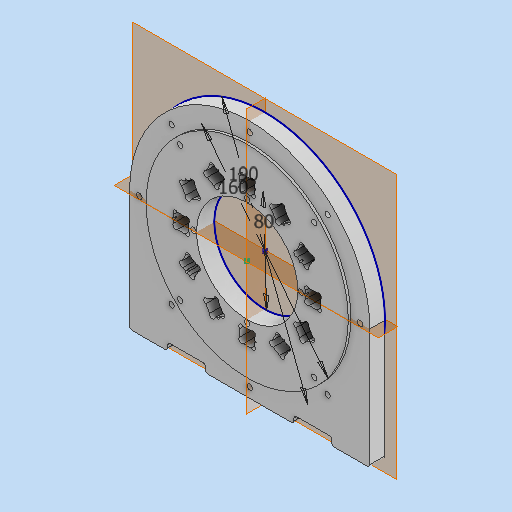
# Autodesk Inventor part: Ring 42 final
Saved by Autodesk Inventor 2026 (Build 300175050, 175E)
## iProperties
Created: 2025-09-01
Part Number: Ring 42 final
Material: Generic
Document SubType Name: Modeling
Designer: user
Density: 1 g/cm^3
Appearance: Default
Author: user
Autodesk Inventor part; units mm, degrees
sketch "Block1" plane through (0, 0, 0) normal (0, 0, 1) x (1, 0, 0)
  line L0 (58.086, -5.94) -> (46.206, -5.94)
  line L1 (46.206, -5.94) -> (46.206, 5.94)
  line L2 (46.206, 5.94) -> (58.086, 5.94)
  line L3 (58.086, 5.94) -> (58.086, -5.94)
  circle A0 centre (47.619, -4.527) radius 2.1
  circle A1 centre (47.619, 4.527) radius 2.1
  circle A2 centre (56.673, 4.527) radius 2.1
  circle A3 centre (56.673, -4.527) radius 2.1
  circle A4 centre (52.146, 0) radius 2
  circle A5 centre (45.846, 0) radius 0.75
  line L4 (45.846, 0) -> (52.146, 0)
  point P0 (52.146, 0)
  dimension "d10" = 4.2
  dimension "d11" = 4.2
  dimension "d12" = 4.2
  dimension "d13" = 4.2
  dimension "d8" = 11.88
  dimension "d9" = 11.88
  dimension "d15" = 1.413
  dimension "d16" = 1.413
  dimension "d17" = 1.413
  dimension "d18" = 1.413
  dimension "d19" = 4
  dimension "d24" = 4.527
  dimension "d25" = 4.527
  dimension "d26" = 1.5
  dimension "d27" = 6.3
  measures "d8" distance of point (46.206, 5.94) point (58.086, 5.94)
  measures "d9" distance of point (58.086, 5.94) point (58.086, -5.94)
  measures "d19" diameter of A4
  measures "d24" horizontal distance of point (56.673, 4.527) L4.end
  measures "d25" horizontal distance of point (47.619, 4.527) L4.end
  measures "d26" diameter of A5
  measures "d27" distance of L4.end L4.start
sketch "Sketch1" plane through (0, 0, 0) normal (0, 0, 1) x (1, 0, 0)
  circle A0 centre (0, 0) radius 40
  circle A1 centre (0, 0) radius 80
  circle A2 centre (0, 0) radius 95
  dimension "d0" = 80
  dimension "d1" = 160
  dimension "d2" = 190
  constraints: 3 centre point, 3 coincident
  measures "d0" diameter of A0
  measures "d1" diameter of A1
  measures "d2" diameter of A2
extrude "Extrusion1" add sketch "Sketch1" along normal blind 14 contours A1
extrude "Extrusion2" add sketch "Sketch1" along normal blind 12 contours A2
sketch "Sketch2" plane through (0, 0, 0) normal (0, 1, 0) x (-1, 0, 0)
  point P0 (0, 0)
sketch "Sketch3" plane through (0, 0, 14) normal (0, 0, 1) x (1, 0, 0)
  point P0 (0, 0)
sketch "Sketch4" plane through (0, 0, 14) normal (0, 0, 1) x (1, 0, 0)
  circle A0 centre (0, 0) radius 52.146
  line L0 (58.086, -5.94) -> (46.206, 5.94) construction
  line L1 (46.206, -5.94) -> (58.086, 5.94) construction
  line L2 (0, 0) -> (52.146, 0)
  line L3 (0, 0) -> (45.1598, 26.073)
  line L4 (0, 0) -> (26.073, 45.1598)
  line L5 (0, 0) -> (0, 52.146)
  line L6 (0, 0) -> (-26.073, 45.1598)
  line L7 (0, 0) -> (-45.1598, 26.073)
  line L8 (0, 0) -> (-52.146, 0)
  line L9 (0, 0) -> (-45.1598, -26.073)
  line L10 (0, 0) -> (-26.073, -45.1598)
  line L11 (0, 0) -> (0, -52.146)
  line L12 (0, 0) -> (26.073, -45.1598)
  line L13 (0, 0) -> (45.1598, -26.073)
  line L14 (58.086, -5.94) -> (46.206, -5.94)
  line L15 (46.206, -5.94) -> (46.206, 5.94)
  line L16 (46.206, 5.94) -> (58.086, 5.94)
  line L17 (58.086, 5.94) -> (58.086, -5.94)
  circle A1 centre (47.619, -4.527) radius 2.1
  circle A2 centre (47.619, 4.527) radius 2.1
  circle A3 centre (56.673, 4.527) radius 2.1
  circle A4 centre (56.673, -4.527) radius 2.1
  circle A5 centre (52.146, 0) radius 2
  circle A6 centre (45.846, 0) radius 0.75
  line L18 (45.846, 0) -> (52.146, 0)
  line L19 (58.086, -5.94) -> (46.206, -5.94)
  line L20 (46.206, -5.94) -> (46.206, 5.94)
  line L21 (46.206, 5.94) -> (58.086, 5.94)
  line L22 (58.086, 5.94) -> (58.086, -5.94)
  circle A7 centre (47.619, -4.527) radius 2.1
  circle A8 centre (47.619, 4.527) radius 2.1
  circle A9 centre (56.673, 4.527) radius 2.1
  circle A10 centre (56.673, -4.527) radius 2.1
  circle A11 centre (52.146, 0) radius 2
  circle A12 centre (45.846, 0) radius 0.75
  line L23 (45.846, 0) -> (52.146, 0)
  line L24 (53.274, 28.2472) -> (47.334, 17.9588)
  line L25 (47.334, 17.9588) -> (37.0456, 23.8988)
  line L26 (37.0456, 23.8988) -> (42.9856, 34.1872)
  line L27 (42.9856, 34.1872) -> (53.274, 28.2472)
  circle A13 centre (46.8168, 19.889) radius 2.1
  circle A14 centre (38.9758, 24.416) radius 2.1
  circle A15 centre (43.5028, 32.257) radius 2.1
  circle A16 centre (51.3438, 27.73) radius 2.1
  circle A17 centre (45.1598, 26.073) radius 2
  circle A18 centre (42.0098, 20.617) radius 0.75
  line L28 (42.0098, 20.617) -> (45.1598, 26.073)
  line L29 (28.2472, 53.274) -> (34.1872, 42.9856)
  line L30 (34.1872, 42.9856) -> (23.8988, 37.0456)
  line L31 (23.8988, 37.0456) -> (17.9588, 47.334)
  line L32 (17.9588, 47.334) -> (28.2472, 53.274)
  circle A19 centre (32.257, 43.5028) radius 2.1
  circle A20 centre (24.416, 38.9758) radius 2.1
  circle A21 centre (19.889, 46.8168) radius 2.1
  circle A22 centre (27.73, 51.3438) radius 2.1
  circle A23 centre (26.073, 45.1598) radius 2
  circle A24 centre (29.223, 39.7038) radius 0.75
  line L33 (29.223, 39.7038) -> (26.073, 45.1598)
  line L34 (-5.94, 58.086) -> (5.94, 58.086)
  line L35 (5.94, 58.086) -> (5.94, 46.206)
  line L36 (5.94, 46.206) -> (-5.94, 46.206)
  line L37 (-5.94, 46.206) -> (-5.94, 58.086)
  circle A25 centre (4.527, 56.673) radius 2.1
  circle A26 centre (4.527, 47.619) radius 2.1
  circle A27 centre (-4.527, 47.619) radius 2.1
  circle A28 centre (-4.527, 56.673) radius 2.1
  circle A29 centre (0, 52.146) radius 2
  circle A30 centre (6.3, 52.146) radius 0.75
  line L38 (6.3, 52.146) -> (0, 52.146)
  line L39 (-34.1872, 42.9856) -> (-28.2472, 53.274)
  line L40 (-28.2472, 53.274) -> (-17.9588, 47.334)
  line L41 (-17.9588, 47.334) -> (-23.8988, 37.0456)
  line L42 (-23.8988, 37.0456) -> (-34.1872, 42.9856)
  circle A31 centre (-27.73, 51.3438) radius 2.1
  circle A32 centre (-19.889, 46.8168) radius 2.1
  circle A33 centre (-24.416, 38.9758) radius 2.1
  circle A34 centre (-32.257, 43.5028) radius 2.1
  circle A35 centre (-26.073, 45.1598) radius 2
  circle A36 centre (-22.923, 50.6157) radius 0.75
  line L43 (-22.923, 50.6157) -> (-26.073, 45.1598)
  line L44 (-47.334, 17.9588) -> (-53.274, 28.2472)
  line L45 (-53.274, 28.2472) -> (-42.9856, 34.1872)
  line L46 (-42.9856, 34.1872) -> (-37.0456, 23.8988)
  line L47 (-37.0456, 23.8988) -> (-47.334, 17.9588)
  circle A37 centre (-51.3438, 27.73) radius 2.1
  circle A38 centre (-43.5028, 32.257) radius 2.1
  circle A39 centre (-38.9758, 24.416) radius 2.1
  circle A40 centre (-46.8168, 19.889) radius 2.1
  circle A41 centre (-45.1598, 26.073) radius 2
  circle A42 centre (-48.3098, 31.529) radius 0.75
  line L48 (-48.3098, 31.529) -> (-45.1598, 26.073)
  line L49 (-37.0456, -23.8988) -> (-42.9856, -34.1872)
  line L50 (-42.9856, -34.1872) -> (-53.274, -28.2472)
  line L51 (-53.274, -28.2472) -> (-47.334, -17.9588)
  line L52 (-47.334, -17.9588) -> (-37.0456, -23.8988)
  circle A43 centre (-43.5028, -32.257) radius 2.1
  circle A44 centre (-51.3438, -27.73) radius 2.1
  circle A45 centre (-46.8168, -19.889) radius 2.1
  circle A46 centre (-38.9758, -24.416) radius 2.1
  circle A47 centre (-45.1598, -26.073) radius 2
  circle A48 centre (-48.3098, -31.529) radius 0.75
  line L53 (-48.3098, -31.529) -> (-45.1598, -26.073)
  line L54 (-23.8988, -37.0456) -> (-17.9588, -47.334)
  line L55 (-17.9588, -47.334) -> (-28.2472, -53.274)
  line L56 (-28.2472, -53.274) -> (-34.1872, -42.9856)
  line L57 (-34.1872, -42.9856) -> (-23.8988, -37.0456)
  circle A49 centre (-19.889, -46.8168) radius 2.1
  circle A50 centre (-27.73, -51.3438) radius 2.1
  circle A51 centre (-32.257, -43.5028) radius 2.1
  circle A52 centre (-24.416, -38.9758) radius 2.1
  circle A53 centre (-26.073, -45.1598) radius 2
  circle A54 centre (-22.923, -50.6157) radius 0.75
  line L58 (-22.923, -50.6157) -> (-26.073, -45.1598)
  line L59 (17.9588, -47.334) -> (23.8988, -37.0456)
  line L60 (23.8988, -37.0456) -> (34.1872, -42.9856)
  line L61 (34.1872, -42.9856) -> (28.2472, -53.274)
  line L62 (28.2472, -53.274) -> (17.9588, -47.334)
  circle A55 centre (24.416, -38.9758) radius 2.1
  circle A56 centre (32.257, -43.5028) radius 2.1
  circle A57 centre (27.73, -51.3438) radius 2.1
  circle A58 centre (19.889, -46.8168) radius 2.1
  circle A59 centre (26.073, -45.1598) radius 2
  circle A60 centre (29.223, -39.7038) radius 0.75
  line L63 (29.223, -39.7038) -> (26.073, -45.1598)
  line L64 (42.9856, -34.1872) -> (37.0456, -23.8988)
  line L65 (37.0456, -23.8988) -> (47.334, -17.9588)
  line L66 (47.334, -17.9588) -> (53.274, -28.2472)
  line L67 (53.274, -28.2472) -> (42.9856, -34.1872)
  circle A61 centre (38.9758, -24.416) radius 2.1
  circle A62 centre (46.8168, -19.889) radius 2.1
  circle A63 centre (51.3438, -27.73) radius 2.1
  circle A64 centre (43.5028, -32.257) radius 2.1
  circle A65 centre (45.1598, -26.073) radius 2
  circle A66 centre (42.0098, -20.617) radius 0.75
  line L68 (42.0098, -20.617) -> (45.1598, -26.073)
  line L69 (-5.94, -46.206) -> (5.94, -46.206)
  line L70 (5.94, -46.206) -> (5.94, -58.086)
  line L71 (5.94, -58.086) -> (-5.94, -58.086)
  line L72 (-5.94, -58.086) -> (-5.94, -46.206)
  circle A67 centre (4.527, -47.619) radius 2.1
  circle A68 centre (4.527, -56.673) radius 2.1
  circle A69 centre (-4.527, -56.673) radius 2.1
  circle A70 centre (-4.527, -47.619) radius 2.1
  circle A71 centre (0, -52.146) radius 2
  circle A72 centre (6.3, -52.146) radius 0.75
  line L73 (6.3, -52.146) -> (0, -52.146)
  line L74 (-46.206, -5.94) -> (-58.086, -5.94)
  line L75 (-58.086, -5.94) -> (-58.086, 5.94)
  line L76 (-58.086, 5.94) -> (-46.206, 5.94)
  line L77 (-46.206, 5.94) -> (-46.206, -5.94)
  circle A73 centre (-56.673, -4.527) radius 2.1
  circle A74 centre (-56.673, 4.527) radius 2.1
  circle A75 centre (-47.619, 4.527) radius 2.1
  circle A76 centre (-47.619, -4.527) radius 2.1
  circle A77 centre (-52.146, 0) radius 2
  circle A78 centre (-58.446, 0) radius 0.75
  line L78 (-58.446, 0) -> (-52.146, 0)
  point P0 (52.146, 0)
  point P1 (-22.4156, -39.6147)
  point P2 (-26.4679, -38.5288)
  point P3 (-31.6181, -41.5023)
  point P4 (-32.7039, -45.5547)
  point P5 (-29.7305, -50.7049)
  point P6 (-25.6781, -51.7907)
  point P7 (-20.5279, -48.8172)
  point P8 (-19.4421, -44.7649)
  point P9 (-2.9735, -46.206)
  point P10 (-5.94, -49.1725)
  point P11 (-5.94, -55.1195)
  point P12 (-2.9735, -58.086)
  point P13 (2.9735, -58.086)
  point P14 (5.94, -55.1195)
  point P15 (5.94, -49.1725)
  point P16 (2.9735, -46.206)
  point P17 (31.6181, -41.5023)
  point P18 (26.4679, -38.5288)
  point P19 (22.4156, -39.6147)
  point P20 (19.4421, -44.7649)
  point P21 (20.5279, -48.8172)
  point P22 (25.6781, -51.7907)
  point P23 (29.7305, -50.7049)
  point P24 (32.7039, -45.5547)
  point P25 (39.6147, -22.4156)
  point P26 (38.5288, -26.4679)
  point P27 (41.5023, -31.6181)
  point P28 (45.5547, -32.7039)
  point P29 (50.7049, -29.7305)
  point P30 (51.7907, -25.6781)
  point P31 (48.8172, -20.5279)
  point P32 (44.7649, -19.4421)
  point P33 (49.1725, 5.94)
  point P34 (46.206, 2.9735)
  point P35 (46.206, -2.9735)
  point P36 (49.1725, -5.94)
  point P37 (55.1195, -5.94)
  point P38 (58.086, -2.9735)
  point P39 (58.086, 2.9735)
  point P40 (55.1195, 5.94)
  point P41 (39.6147, 22.4156)
  point P42 (44.7649, 19.4421)
  point P43 (48.8172, 20.5279)
  point P44 (51.7907, 25.6781)
  point P45 (50.7049, 29.7305)
  point P46 (45.5547, 32.7039)
  point P47 (41.5023, 31.6181)
  point P48 (38.5288, 26.4679)
  point P49 (20.5279, 48.8172)
  point P50 (19.4421, 44.7649)
  point P51 (22.4156, 39.6147)
  point P52 (26.4679, 38.5288)
  point P53 (31.6181, 41.5023)
  point P54 (32.7039, 45.5547)
  point P55 (29.7305, 50.7049)
  point P56 (25.6781, 51.7907)
  point P57 (-5.94, 49.1725)
  point P58 (-2.9735, 46.206)
  point P59 (2.9735, 46.206)
  point P60 (5.94, 49.1725)
  point P61 (5.94, 55.1195)
  point P62 (2.9735, 58.086)
  point P63 (-2.9735, 58.086)
  point P64 (-5.94, 55.1195)
  point P65 (-20.5279, 48.8172)
  point P66 (-25.6781, 51.7907)
  point P67 (-29.7305, 50.7049)
  point P68 (-32.7039, 45.5547)
  point P69 (-31.6181, 41.5023)
  point P70 (-26.4679, 38.5288)
  point P71 (-22.336, 38.687)
  point P72 (-22.6435, 39.2198)
  point P73 (-19.4421, 44.7649)
  point P74 (-44.7649, 19.4421)
  point P75 (-39.6147, 22.4156)
  point P76 (-38.5288, 26.4679)
  point P77 (-41.5023, 31.6181)
  point P78 (-45.5547, 32.7039)
  point P79 (-50.7049, 29.7305)
  point P80 (-51.7907, 25.6781)
  point P81 (-48.8172, 20.5279)
  point P82 (-49.1725, -5.94)
  point P83 (-46.206, -2.9735)
  point P84 (-46.206, 2.9735)
  point P85 (-49.1725, 5.94)
  point P86 (-55.1195, 5.94)
  point P87 (-58.086, 2.9735)
  point P88 (-58.086, -2.9735)
  point P89 (-55.1195, -5.94)
  point P90 (-48.8172, -20.5279)
  point P91 (-51.7907, -25.6781)
  point P92 (-50.7049, -29.7305)
  point P93 (-48.6996, -30.8882)
  point P94 (-47.56, -31.5462)
  point P95 (-45.5547, -32.7039)
  point P96 (-41.5314, -31.5333)
  point P97 (-41.487, -31.5917)
  point P98 (-38.5288, -26.4679)
  point P99 (-39.6147, -22.4156)
  point P100 (-44.7649, -19.4421)
  dimension "d7" = 104.292
  dimension "d28" = 52.146
  dimension "d31" = 360
  dimension "d33" = 0
  dimension "d34" = -60
  dimension "d35" = -120
  dimension "d36" = -180
  dimension "d37" = -180
  dimension "d38" = -240
  dimension "d39" = -300
  dimension "d40" = -60
  dimension "d41" = -120
  dimension "d42" = -180
  dimension "d43" = -240
  dimension "d44" = -240
  constraints: 28 end point, 2 midpoint, 1 centre point, 1 coincident, 1 horizontal, 57 other
  measures "d7" diameter of A0
  measures "d28" distance of point (52.146, 0) point (0, 0)
  measures "d33" vertical extent of L2
  measures "d36" angle to the sketch x axis of L2
  measures "d37" angle to the sketch x axis of L8
  measures "d42" angle to the sketch x axis of L8
extrude "Extrusion3" cut sketch "Sketch4" against normal blind 12 contours L2 A5 A0 | A0 A5 | A0 A5 L2 | A5 L2 A6 L15 A2 L16 A0 | A0 L16 A3 L17 A4 L14 A5 | A0 L14 A1 L15 A6 L2 A5 | A6 L15 L2 | L2 L15 A6 | A13 L25 L24 A0 | A0 L24 A13 | A2 L15 L16 | L16 L15 A2 | A3 L17 L16 | L16 L17 A3 | A62 L66 A0 | A0 L66 L65 A62 | A4 L17 L14 | L14 L17 A4 | A1 L15 L14 | L14 L15 A1 | L24 L25 A13 A0 | A0 A13 L24 | L25 A18 L28 A17 A0 A13 | L66 A62 A0 | A0 A62 L65 L66 | A62 A0 A65 L68 A66 L65 | A0 A17 A15 L27 A16 L24 A13 | L25 L28 A18 | A62 L66 A63 L67 A64 A0 A65 | A66 L68 L65 | A17 L28 A0 | A0 A17 | A16 L27 L24 | L24 L27 A16 | L25 A18 L28 | L25 A14 L3 A17 L28 A18 | A65 A0 | A0 L68 A65 | A63 L67 L66 | L66 L67 A63 | L68 A66 L65 | A66 L68 A65 L13 A61 L65 | A14 L26 L25 L3 | L3 L25 A14 | A20 L31 L4 | L4 L31 L30 A20 | L36 A27 L37 A0 A29 L5 | L5 A29 A0 A30 L35 A26 L36 | A33 L42 L41 L6 | A39 L47 L7 | L7 L47 L46 A39 | L77 A76 L74 A0 A77 L8 | L8 A77 A0 L76 A75 L77 | A46 L49 L52 L9 | L9 L52 A46 | A52 L54 L10 | L10 L54 L57 A52 | L69 A67 L70 A72 A0 A71 L11 | L11 A71 A0 L72 A70 L69 | A55 L60 L59 L12 | L12 L59 A55 | A61 L65 L13 | L13 L65 L64 A61 | L3 A17 A0 | L28 A17 L3 | L25 L3 A14 | A0 A65 L13 | L13 A65 L68 | A61 L13 L65 | L25 L26 A14 L3 | L26 A0 A15 A17 L3 A14 | L31 A20 L4 | L4 A20 L30 L31 | L31 A21 A0 A23 L4 A20 | A20 L4 A23 L33 A24 L30 | A29 A0 L5 | L5 A0 A29 | A26 L35 L36 | L36 L35 A26 | A27 L37 L36 | L36 L37 A27 | L41 L42 A33 L6 | L6 A33 L41 | L42 A0 A34 A35 L6 A33 | L47 A39 L7 | L7 A39 L46 L47 | L47 A40 A0 A41 L7 A39 | A77 A0 L8 | L8 A0 A77 | A75 L76 L77 | L77 L76 A75 | A76 L74 L77 | L77 L74 A76 | L52 L49 A46 L9 | L9 A46 L52 | A46 L9 A47 A0 A45 L52 | L54 A52 L10 | L10 A52 L57 L54 | A52 L10 A53 A0 A51 L57 | A71 A0 L11 | L11 A0 A71 | A70 L72 L69 | L69 L72 A70 | A67 L70 L69 | L69 L70 A67 | L59 L60 A55 L12 | L12 A55 L59 | L60 A60 L63 A59 L12 A55 | A55 L12 A59 A0 A58 L59 | L13 A61 L64 L65 | A61 L13 A65 A0 A64 L64 | A15 A0 L26 L27 | L27 L26 A15 | A64 L64 L67 | L67 L64 A64 A0 | L26 A15 A0 | A21 A0 L32 L31 | L31 L32 A0 A21 | A24 L33 L30 | L38 A29 A0 | A0 A29 L38 | A0 L37 A28 L34 A25 L35 A30 L38 A29 | A29 L38 A30 A0 | L6 A35 A0 A32 L41 A33 | L42 A34 A0 | L7 A41 A0 A38 L46 A39 | A40 A0 L44 L47 | L47 L44 A0 A40 | L78 A77 A0 | A0 A77 L78 | A77 L78 A78 L75 A74 L76 A0 | A0 L74 A73 L75 A78 L78 A77 | A46 L49 A0 A43 A47 L9 | A45 A0 L51 L52 | L52 L51 A0 A45 | A52 L54 A49 A0 A53 L10 | A0 A51 L57 | L73 A71 A0 | A0 A71 L73 | A0 A72 L73 A71 | A71 L73 A72 L70 A68 L71 A69 L72 A0 | L60 L63 A60 | A58 A0 L62 L59 | L59 L62 A0 A58 | A0 A64 L64 | A15 A0 | A0 A64 | L30 A24 L33 A23 A0 A19 | A0 A19 L30 | A23 A0 L4 | L4 L33 A23 | A21 L32 A0 | L33 A24 L30 | A30 L38 L35 A0 | A0 L35 A30 | A35 A0 L6 | L6 A0 A35 | A32 A0 L40 L41 | L41 L40 A0 A32 | A34 L42 L39 A0 | A0 A34 | A0 A38 L46 | A34 L39 L42 | A41 A0 L7 | L7 A0 A41 | A40 L44 A0 | A47 A0 L9 | L9 A0 A47 | A0 L51 A45 | A53 A0 L10 | L10 A0 A53 | A49 A0 L55 L54 | L54 L55 A0 A49 | A51 A0 | A0 A51 L56 L57 | L57 L56 A51 | A72 L70 A0 | A0 L70 L73 A72 | A59 L63 L12 | L12 A0 A59 | L60 A60 L63 | A60 L60 A0 A56 A59 L63 | A0 L62 A58 | L60 A56 A0 | A19 A0 | A0 A19 L29 L30 | L30 L29 A19 | A0 A23 | A0 A23 L33 | A0 A21 L32 A22 L29 A19 A23 | L32 A21 A0 | A30 L35 L38 | A0 L40 A32 | A28 L34 L37 | L37 L34 A28 | L43 A35 A0 | A0 A35 L43 | A0 A34 L39 A31 L40 A36 L43 A35 | A32 L40 A0 | A0 A35 L43 A36 L40 A32 | A38 A0 | A0 A38 L45 L46 | L46 L45 A38 | L48 A41 A0 | A0 A41 L48 | A0 A40 L44 A37 L45 A42 L48 A41 | L44 A40 A0 | L78 L75 A78 | A78 L75 L78 | A74 L75 L76 | L76 L75 A74 | A73 L75 L74 | L74 L75 A73 | L53 A47 A0 | A0 A47 L53 | A47 L53 A48 L50 A44 L51 A45 A0 | A43 L49 L50 A0 | A0 A43 | A43 L50 L49 | A0 A45 L51 | L58 A53 A0 | A0 A53 L58 | A53 L58 A54 L55 A50 L56 A51 A0 | A49 L55 A54 L58 A53 A0 | A0 L55 A49 | L73 L70 A72 | A49 L55 A0 | A69 L71 L72 | L72 L71 A69 | A0 A59 | L63 A59 A0 | A59 A0 A56 L61 A57 L62 A58 | A0 A58 L62 | A56 L60 L61 A0 | A0 A56 | A56 L61 L60 | A22 L29 L32 | L32 L29 A22 | A0 A41 L48 A42 L45 A38 | A31 L40 L39 | L39 L40 A31 | A37 L45 L44 | L44 L45 A37 | A0 A43 L50 A48 L53 A47 | A44 L50 L51 | L51 L50 A44 | A50 L55 L56 | L56 L55 A50 | A57 L61 L62 | L62 L61 A57 | A25 L34 L35 | L35 L34 A25 | A36 L43 L40 | A36 L40 L43 | L48 L45 A42 | A42 L45 L48 | L58 L55 A54 | A54 L55 L58 | A68 L71 L70 | L70 L71 A68 picked at (46.2498, -0.4081) picked at (46.2498, 0.4081) picked at (-23.1639, 40.2816) picked at (5.8954, 51.6254) picked at (5.8954, -51.6254)
extrude "Extrusion4" cut sketch "Sketch4" against normal blind 2 contours A6 L15 L2 | L2 L15 A6 | L15 A6 L2 | L2 A6 L15 | A18 L25 | L25 L28 A18 | A66 L68 L65 | L65 A66 | L25 A18 L28 | L68 A66 L65 | A24 L33 L30 | L30 A24 | A60 L60 | L60 L63 A60 | L33 A24 L30 | A30 L38 L35 A0 | A0 L35 A30 | L35 A0 A30 | A72 L70 A0 | A0 L70 L73 A72 | A72 A0 L70 | L60 A60 L63 | A0 L35 A30 | A30 L35 L38 | L78 L75 A78 | A78 L75 L78 | L73 L70 A72 | A0 A72 L70 | L75 A78 | A36 L43 L40 | L40 A36 | A36 L40 L43 | L48 L45 A42 | A42 L45 L48 | L53 L50 A48 | A48 L50 L53 | L58 L55 A54 | A54 L55 L58 | A54 L55 | L45 A42 | L50 A48
extrude "Extrusion5" cut sketch "Sketch4" against normal through all contours L2 A5 A0 | A0 A5 | A0 A5 L2 | A17 L28 A0 | A0 A17 | A65 A0 | A0 L68 A65 | L3 A17 A0 | L28 A17 L3 | A0 A65 L13 | L13 A65 L68 | A29 A0 L5 | L5 A0 A29 | A77 A0 L8 | L8 A0 A77 | A71 A0 L11 | L11 A0 A71 | L38 A29 A0 | A0 A29 L38 | L78 A77 A0 | A0 A77 L78 | L73 A71 A0 | A0 A71 L73 | A23 A0 L4 | L4 L33 A23 | A35 A0 L6 | L6 A0 A35 | A41 A0 L7 | L7 A0 A41 | A47 A0 L9 | L9 A0 A47 | A59 L63 L12 | L12 A0 A59 | A0 A23 | A0 A23 L33 | L43 A35 A0 | A0 A35 L43 | L48 A41 A0 | A0 A41 L48 | L53 A47 A0 | A0 A47 L53 | A0 A59 | L63 A59 A0
extrude "Extrusion6" cut sketch "Sketch4" against normal through all contours A53 A0 L10 | L10 A0 A53 | L58 A53 A0 | A0 A53 L58
sketch "Sketch5" plane through (0, 0, 12) normal (0, 0, 1) x (1, 0, 0)
  circle A0 centre (87.25, 0) radius 2.15
  circle A1 centre (61.6951, 61.6951) radius 2.15
  circle A2 centre (0, 87.25) radius 2.15
  circle A3 centre (-61.6951, 61.6951) radius 2.15
  circle A4 centre (-87.25, 0) radius 2.15
  circle A5 centre (-61.6951, -61.6951) radius 2.15
  circle A6 centre (0, -87.25) radius 2.15
  circle A7 centre (61.6951, -61.6951) radius 2.15
  point P0 (0, 0)
  dimension "d53" = 4.3
  dimension "d54" = 87.25
  dimension "d57" = 360
  constraints: 8 centre point, 17 other
  measures "d53" diameter of A0
  measures "d54" distance of A0.centre point (0, 0)
extrude "Extrusion7" cut sketch "Sketch5" against normal through all
sketch "Sketch6" plane through (0, 0, 14) normal (0, 0, 1) x (1, 0, 0)
  circle A0 centre (0, 0) radius 42.5
  circle A1 centre (42.5, 0) radius 2.1
  circle A2 centre (0, 42.5) radius 2.1
  circle A3 centre (-42.5, 0) radius 2.1
  circle A4 centre (0, -42.5) radius 2.1
  dimension "d61" = 85
  dimension "d62" = 4.2
  dimension "d65" = 360
  constraints: 4 centre point, 1 coincident, 1 horizontal alignment, 11 other
  measures "d62" diameter of A1
extrude "Extrusion8" cut sketch "Sketch6" against normal blind 10 contours A0 A1 | A0 A1 | A2 A0 | A0 A2 | A4 A0 | A0 A4 | A3 A0 | A0 A3
sketch "Sketch7" plane through (0, 0, 14) normal (0, 0, 1) x (1, 0, 0)
  point P0 (0, 0)
sketch "Sketch8" plane through (0, 0, 14) normal (0, 0, 1) x (1, 0, 0)
  circle A0 centre (0, 0) radius 75
  circle A1 centre (53.033, 53.033) radius 2.1
  line L0 (53.033, 53.033) -> (0, 0)
  line L1 (-133, 0) -> (133, 0) projected
  circle A2 centre (-53.033, 53.033) radius 2.1
  circle A3 centre (-53.033, -53.033) radius 2.1
  circle A4 centre (53.033, -53.033) radius 2.1
  dimension "d69" = 150
  dimension "d70" = 4.2
  dimension "d71" = 45
  dimension "d74" = 360
  constraints: 4 centre point, 2 end point, 1 coincident, 12 other
  measures "d70" diameter of A1
  measures "d71" angle of L1 L0
extrude "Extrusion9" cut sketch "Sketch8" against normal blind 10 contours A1 L0 A0 | A0 A1 | A4 A0 | A0 A4 | L0 A1 A0 | A3 A0 | A0 A3 | A2 A0 | A0 A2
sketch "Sketch9" plane through (0, 0, 0) normal (0, 0, 1) x (1, 0, 0)
  circle A0 centre (0, 0) radius 95 projected
  line L0 (-95, 0) -> (-95, -95)
  line L1 (-95, -95) -> (95, -95)
  line L2 (95, -95) -> (95, 0)
  line L3 (-65, -89) -> (-35, -89)
  line L4 (-35, -89) -> (-35, -101)
  line L5 (-35, -101) -> (-65, -101)
  line L6 (-65, -101) -> (-65, -89)
  line L7 (-65, -89) -> (-35, -101) construction
  line L8 (-35, -89) -> (-65, -101) construction
  line L9 (35, -89) -> (65, -89)
  line L10 (65, -89) -> (65, -101)
  line L11 (65, -101) -> (35, -101)
  line L12 (35, -101) -> (35, -89)
  line L13 (35, -89) -> (65, -101) construction
  line L14 (65, -89) -> (35, -101) construction
  point P0 (-50, -95)
  point P1 (50, -95)
  point P2 (0, -95)
  point P3 (35, -95)
  point P4 (65, -95)
  point P5 (-35, -95)
  point P6 (-65, -95)
  dimension "d78" = 30
  dimension "d79" = 12
  dimension "d81" = 45
  dimension "d82" = 95
  dimension "d83" = 190
  dimension "d84" = 30
  dimension "d85" = 45
  dimension "d86" = 12
  constraints: 30 end point, 4 midpoint, 4 parallel, 3 perpendicular, 2 horizontal, 2 point on circle, 2 point on line, 2 tangent, 1 vertical
  measures "d78" distance of L4.end L5.end
  measures "d79" distance of L3.end L4.end
  measures "d81" distance of point (-50, -95) L0.end
  measures "d82" distance of L1.end L2.end
  measures "d83" distance of L0.end L1.end
  measures "d84" distance of L10.end L11.end
  measures "d85" distance of point (50, -95) L1.end
  measures "d86" distance of L10.end L9.end
extrude "Extrusion10" add sketch "Sketch9" along normal blind 12 contours L2 L1 L10 L9 L12 A0 | A0 L1 L4 L3 L6 L0
fillet "Fillet1" radius 2 10 edges at (-35, -89, 6) (65, -89, 6) (-65, -89, 6) (35, -89, 6) (35, -95, 6) (-35, -95, 6) (-65, -95, 6) (-95, -95, 6) (95, -95, 6) (65, -95, 6)
body "Solid1"
